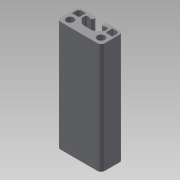
# Autodesk Inventor part: 40-4020
Saved by Autodesk Inventor 2013 (Build 170138000, 138)
## iProperties
Created: 2014-04-23
Part Number: 40-4020
Material: Generic
Document SubType Name: Modeling
Designer: Ross Bowman
Density: 1 g/cm^3
Engineer: Ross Bowman
Catalog Web Link: 8020.net
Vendor: 80/20 Inc.
Company: 80/20 Inc.
Author: Ross Bowman
Keywords: 80/20 , 8020 , T-Slot , Extrusion
Material: 6105-T5 Aluminum
Autodesk Inventor part; units mm, degrees
ref_plane "YZ Plane" through (0, 0, 0) normal (1, 0, 0) x (0, 1, 0)
ref_plane "XZ Plane" through (0, 0, 0) normal (0, 1, 0) x (-1, 0, 0)
ref_plane "XY Plane" through (0, 0, 0) normal (0, 0, 1) x (1, 0, 0)
sketch "Sketch1" plane through (0, 0, 0) normal (0, 0, 1) x (1, 0, 0)
  arc A0 (17.687, 1.9459) -> (18.324, 2.5123) centre (17.6928, 2.5809) ccw
  line L0 (13.2104, 1.9459) -> (17.687, 1.9459)
  arc A1 (11.9404, 3.2159) -> (13.2104, 1.9459) centre (13.2104, 3.2159) ccw
  line L1 (11.9404, 7.6925) -> (11.9404, 3.2159)
  arc A2 (12.5686, 8.3275) -> (11.9404, 7.6925) centre (12.5754, 7.6925) ccw
  line L2 (15.5601, 8.3275) -> (12.5686, 8.3275)
  arc A3 (18.324, 5.5037) -> (15.5601, 8.3275) centre (15.5302, 5.5336) ccw
  line L3 (18.324, 2.5123) -> (18.324, 5.5037)
  circle A4 centre (14, -4) radius 3.4036
  circle A5 centre (-14, -4) radius 3.4036
  arc A6 (-13.2123, 1.9392) -> (-11.9423, 3.2092) centre (-13.2123, 3.2092) ccw
  line L4 (-17.6889, 1.9392) -> (-13.2123, 1.9392)
  arc A7 (-18.3171, 2.5742) -> (-17.6889, 1.9392) centre (-17.6821, 2.5742) ccw
  line L5 (-18.3171, 5.5656) -> (-18.3171, 2.5742)
  arc A8 (-15.4934, 8.3296) -> (-18.3171, 5.5656) centre (-15.5233, 5.5357) ccw
  line L6 (-12.5019, 8.3296) -> (-15.4934, 8.3296)
  arc A9 (-11.9423, 7.6857) -> (-12.5019, 8.3296) centre (-12.5772, 7.6991) ccw
  line L7 (-11.9423, 3.2092) -> (-11.9423, 7.6857)
  arc A10 (-16.825, 10) -> (-20, 6.825) centre (-16.825, 6.825) ccw
  line L8 (-20, 6.825) -> (-20, -6.825)
  arc A11 (-20, -6.825) -> (-16.825, -10) centre (-16.825, -6.825) ccw
  line L9 (-16.825, -10) -> (16.825, -10)
  arc A12 (16.825, -10) -> (20, -6.825) centre (16.825, -6.825) ccw
  line L10 (20, -6.825) -> (20, 6.825)
  arc A13 (20, 6.825) -> (16.825, 10) centre (16.825, 6.825) ccw
  line L11 (16.825, 10) -> (5.6244, 10)
  arc A14 (5.6244, 10) -> (4.06, 8.4356) centre (5.6244, 8.4356) ccw
  line L12 (4.06, 8.4356) -> (4.06, 7.5148)
  arc A15 (4.06, 7.5148) -> (5.6348, 5.94) centre (5.6348, 7.5148) ccw
  line L13 (5.6348, 5.94) -> (6.7718, 5.94)
  line L14 (6.7718, 5.94) -> (6.7718, 6.7089)
  line L15 (6.7718, 6.7089) -> (9.0158, 6.7089)
  arc A16 (10.285, 5.3946) -> (9.0158, 6.7089) centre (9.0158, 5.4389) ccw
  line L16 (10.285, 5.3946) -> (10.285, 3.0962)
  arc A17 (10.1069, 2.5504) -> (10.285, 3.0962) centre (9.3961, 3.0842) ccw
  line L17 (10.1069, 2.5504) -> (6.7378, -0.8187)
  arc A18 (3.3792, -2.3) -> (6.7378, -0.8187) centre (3.2907, 2.449) ccw
  line L18 (3.3792, -2.3) -> (-3.3792, -2.3)
  arc A19 (-6.7378, -0.8187) -> (-3.3792, -2.3) centre (-3.2907, 2.449) ccw
  line L19 (-6.7378, -0.8187) -> (-10.0246, 2.4681)
  arc A20 (-10.285, 3.0967) -> (-10.0246, 2.4681) centre (-9.396, 3.0967) ccw
  line L20 (-10.285, 3.0967) -> (-10.285, 5.3946)
  arc A21 (-9.0158, 6.7089) -> (-10.285, 5.3946) centre (-9.0158, 5.4389) ccw
  line L21 (-9.0158, 6.7089) -> (-6.7718, 6.7089)
  line L22 (-6.7718, 6.7089) -> (-6.7718, 5.94)
  line L23 (-6.7718, 5.94) -> (-5.6348, 5.94)
  arc A22 (-5.6348, 5.94) -> (-4.06, 7.5148) centre (-5.6348, 7.5148) ccw
  line L24 (-4.06, 7.5148) -> (-4.06, 8.4356)
  arc A23 (-4.06, 8.4356) -> (-5.6244, 10) centre (-5.6244, 8.4356) ccw
  line L25 (-5.6244, 10) -> (-16.825, 10)
  point P0 (0, 0)
  constraints: 52 end point, 44 point on circle, 24 centre point
extrude "Extrusion1" add sketch "Sketch1" against normal blind 100
body "Solid1"
